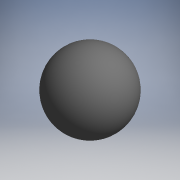
# Autodesk Inventor part: 606 Ball
Saved by Autodesk Inventor 2017.3 (Build 213256000, 256)
## iProperties
Part Number: 606 Ball
Material: Generic
Catalog Web Link: www.cadenas.de
Description: open_type_B-
Vendor: NSK_RB
Document SubType Name: Modeling
Designer: partserver
Manufacturer: NSK_RB
Mass: 0.0188166 g
Surface Area: 0.342119 cm^2
Volume: 0.0188166 cm^3
Density: 1 g/cm^3
Appearance: PSOLRGB-128-128-128
Category: PARTsolutions
Company: NSK_RB
Title: 606 Ball
Author: Cadenas PARTsolutions
PSOL_IDENT_0: {$CADENAS_DATA\23d-libs\nsk_rb\roller_bearings\deep_groove_bb\exstra_small_miniatur_bb\metric_design
PSOL_IDENT_1: \open_type_b.prj},163 {VTYP=3D},{NB=606 Ball},{LINA=606 Ball},{NN=open_type_B},{DATE=10.04.2020 04:5
PSOL_IDENT_2: 7:45},{GEOMDATE=04.01.2008 00:00:00},{VERSION=},{LINEID=1680},{WBVAR=},{WBNUMERIC=}  {NB=606 Ball},{
PSOL_IDENT_3: LINA=606 Ball},{KT=DUMMY},{IDNR=},{STAN=Standard},{ORDER=606},{SD=6.0},{X=6.0},{DI1=8.92},{SDE1=13.7
PSOL_IDENT_4: 5},{D=17},{DD=17},{B=6.0},{B1=0.0},{R=0.30},{R1=0.00},{CR1=2260},{COR1=835},{CR2=231},{COR2=85.0},{L
PSOL_IDENT_5: G=38000},{LO=45000},{DA=8.0},{DB=0.0},{DA1=15.0},{DB1=0.0},{RA=0.30},{RB=0.00},{MASS=5.97},{SC=1}
NB: 606 Ball
NN: open_type_B
NBSYN: $ORDER. Ball
LINA: 606 Ball
CATALOG: NSK Rolling Bearing
STAN: Standard
ORDER: 606
SD: 6
X: 6
DI1: 8.92
SDE1: 13.75
D: 17
DD: 17
B: 6
B1: 0
R: 0.3
R1: 0
CR1: 2260
COR1: 835
CR2: 231
COR2: 85
LG: 38000
LO: 45000
DA: 8
DB: 0
DA1: 15
DB1: 0
RA: 0.3
RB: 0
MASS: 5.97
SC: 1
SUPPLIER: NSK_RB
ARTICLENO: 606 Ball
BOMINFO: 606 Ball
CREATOR: CADENAS GmbH
Autodesk Inventor part; units mm, degrees
ref_plane "YZ Plane" through (0, 0, 0) normal (1, 0, 0) x (0, 1, 0)
ref_plane "XZ Plane" through (0, 0, 0) normal (0, 1, 0) x (-1, 0, 0)
ref_plane "XY Plane" through (0, 0, 0) normal (0, 0, 1) x (1, 0, 0)
sketch "Sketch_1" plane through (0, 0, 0) normal (0, 0, 1) x (1, 0, 0)
  line L0 (1.65, 0) -> (-1.65, 0)
  arc A0 (1.65, 0) -> (-1.65, 0) centre (0, 0) ccw
  line L1 (1.65, 0) -> (-1.65, 0)
  constraints: 4 end point, 2 point on circle, 1 centre point
revolve "Revolution1" add sketch "Sketch_1" angle 360 about axis through (1.65, 0, 0) along (1, 0, 0)
ref_plane "ip_op_b_XY" through (0, 0, 0) normal (-1, 0, 0) x (0, 0, -1)
ref_plane "ip_op_b_YZ" through (0, 0, 0) normal (0, 0, -1) x (0, -1, 0)
ref_plane "ip_op_b_ZX" through (0, 0, 0) normal (0, -1, 0) x (-1, 0, 0)
body "Solid1"
